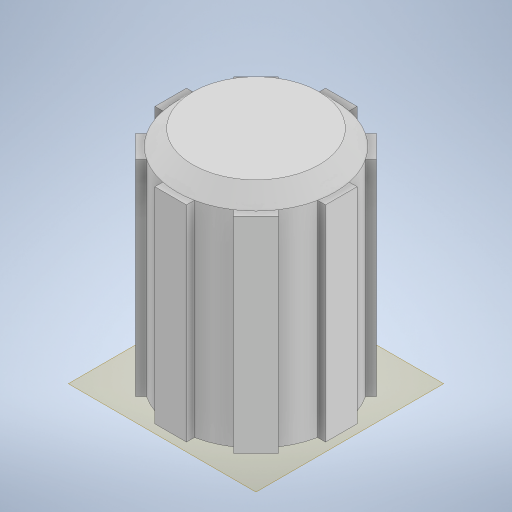
# Autodesk Inventor part: Pot-knob
Saved by Autodesk Inventor 2023 (Build 270158000, 158)
## iProperties
Created: 2023-04-27
Part Number: Pot-knob
Material: Generic
Document SubType Name: Modeling
Designer: ringl
Density: 1 g/cm^3
Appearance: Default
Author: ringl
Autodesk Inventor part; units mm, degrees
ref_plane "YZ Plane" through (0, 0, 0) normal (1, 0, 0) x (0, 1, 0)
ref_plane "XY Plane" through (0, 0, 0) normal (0, 0, 1) x (1, 0, 0)
sketch "Sketch1" plane through (0, 0, 0) normal (0, 1, 0) x (-1, 0, 0)
  arc A0 (1.5, 2.5981) -> (1.5, -2.5981) centre (0, 0) ccw
  line L0 (1.5, 2.5981) -> (1.5, -2.5981)
  line L1 (1.5, 0) -> (-3, 0) construction
  circle A1 centre (0, 0) radius 5
  dimension "d0" = 6
  dimension "d1" = 4.5
  dimension "d2" = 10
  constraints: 4 end point, 3 point on circle, 2 centre point, 2 coincident, 1 horizontal, 1 midpoint, 1 vertical
  measures "d0" diameter of A0
  measures "d1" distance of L1.start L1.end
  measures "d2" diameter of A1
extrude "Extrusion1" add sketch "Sketch1" along normal blind 12
sketch "Sketch2" plane through (0, 12, 0) normal (0, 1, 0) x (1, 0, 0)
  circle A0 centre (0, 0) radius 5
  constraints: 1 centre point, 1 coincident
extrude "Extrusion2" add sketch "Sketch2" along normal blind 2
chamfer "Chamfer1" distance 1 angle 45 1 edges at (-5, 14, 0)
sketch "Sketch3" plane through (0, 0, 0) normal (0, 1, 0) x (-1, 0, 0)
  circle A0 centre (0, 0) radius 5 projected
  line L0 (4.899, 1) -> (5.399, 1)
  line L1 (5.399, 1) -> (5.399, -1)
  line L2 (5.399, -1) -> (4.899, -1)
  arc A1 (4.899, -1) -> (4.899, 1) centre (0, 0) ccw
  dimension "d10" = 2
  dimension "d11" = 0.5
  dimension "d12" = 1
  constraints: 6 end point, 4 point on circle, 2 perpendicular, 1 centre point, 1 concentric, 1 horizontal
  measures "d10" distance of L0.end L1.end
  measures "d11" distance of L1.end L2.end
  measures "d12" distance from line of point (0, 0) L2
extrude "Extrusion3" add sketch "Sketch3" along normal blind 13 contours A0 L0 L1 L2
pattern_circular "Circular Pattern1" count 8 over 360 about axis through (0, 0, 0) along (0, 1, 0) of "Extrusion3"
body "Solid1"
